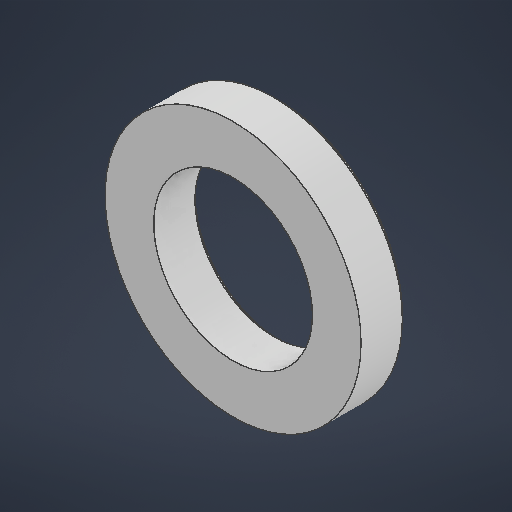
# Autodesk Inventor part: Проставка
Saved by Autodesk Inventor 2025 (Build 290162010, 162A)
## iProperties
Created: 2025-01-30
Part Number: Проставка
Material: Типовые
Document SubType Name: Modeling
Designer: Edward_Higgins
Density: 1 g/cm^3
Appearance: По умолчанию
Author: Edward_Higgins
Autodesk Inventor part; units mm, degrees
ref_plane "YZ Plane" through (0, 0, 0) normal (1, 0, 0) x (0, 1, 0)
ref_plane "XZ Plane" through (0, 0, 0) normal (0, 1, 0) x (-1, 0, 0)
ref_plane "XY Plane" through (0, 0, 0) normal (0, 0, 1) x (1, 0, 0)
sketch "Эскиз1" plane through (0, 0, 0) normal (0, 0, 1) x (1, 0, 0)
  circle A0 centre (0, 0) radius 13.95
  circle A1 centre (0, 0) radius 8.65
  dimension "d0" = 17.3
  dimension "d1" = 27.9
  constraints: 2 centre point, 2 coincident
  measures "d0" diameter of A1
  measures "d1" diameter of A0
extrude "Выдавливание1" add sketch "Эскиз1" along normal blind 5
chamfer "Фаска2" distance 0.5 angle 45 2 edges at (-8.65, 0, 0) (-13.95, 0, 0)
